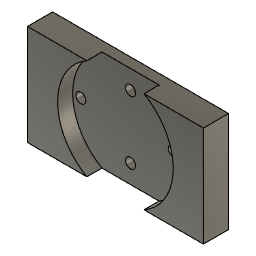
simple_mount v2 (Autodesk Fusion 360 design; units mm, degrees)
Autodesk Fusion 360 part; units mm, degrees
sketch "Sketch1" plane through (0, 0, 0) normal (0, 1, 0) x (1, 0, 0) in component "base_plate"
  line L0 (0, 0) -> (35, 0)
  line L1 (35, 0) -> (35, -20)
  line L2 (0, 0) -> (0, -20)
  line L3 (0, -20) -> (35, -20)
  dimension "d1" = 35
  dimension "d2" = 20
  dimension "d3" = 20
  constraint coincident L0.start L2.start
  constraint horizontal L0
  constraint perpendicular L0 L1
  constraint perpendicular L0 L2
  measures "d1" distance of L0.start L0.end
  measures "d2" distance of L0.end L1.end
  measures "d3" distance of L0.start L2.end
extrude "Extrude1" add sketch "Sketch1" along normal blind 5 in component "base_plate"
sketch "Sketch2" plane through (0, 0, 0) normal (0, -1, 0) x (1, 0, 0) in component "base_plate"
  line L0 (0, 20) -> (0, 0)
  line L1 (0, 0) -> (35, 0)
  line L2 (35, 0) -> (35, 20)
  line L3 (35, 20) -> (0, 20)
  line L4 (0, 10) -> (35, 10) construction
  line L5 (17.5, 20) -> (17.5, 0) construction
  circle A0 centre (7.6246, 10) radius 1
  circle A1 centre (26.0211, 10) radius 1
  dimension "d6" = 2
  dimension "d7" = 2
  constraint midpoint L0 L4.start
  constraint midpoint L2 L4.end
  constraint midpoint L3 L5.start
  constraint perpendicular L4 L5
  constraint coincident L4 A0.centre
  constraint coincident L4 A1.centre
  measures "d6" diameter of A0
  measures "d7" diameter of A1
extrude "Extrude2" cut sketch "Sketch2" against normal blind 5 contours A0 | A1 in component "base_plate"
sketch "Sketch3" plane through (0, 0, 0) normal (0, -1, 0) x (1, 0, 0) in component "base_plate"
  circle A0 centre (7.6246, 10) radius 1
  circle A1 centre (26.0211, 10) radius 1
  line L0 (0, 20) -> (0, 0)
  line L1 (0, 0) -> (35, 0)
  line L2 (35, 0) -> (35, 20)
  line L3 (35, 20) -> (0, 20)
  line L4 (17.5, 20) -> (17.5, 0) construction
  circle A2 centre (17.5, 16.2296) radius 1
  circle A3 centre (17.5, 3.7004) radius 1
  dimension "d10" = 2
  dimension "d11" = 2
  constraint midpoint L3 L4.start
  constraint midpoint L1 L4.end
  constraint coincident L4 A2.centre
  constraint coincident L4 A3.centre
  measures "d10" diameter of A2
  measures "d11" diameter of A3
extrude "Extrude3" cut sketch "Sketch3" against normal blind 5 contours A2 | A3 in component "base_plate"
sketch "Sketch4" plane through (0, 0, 0) normal (0, -1, 0) x (1, 0, 0) in component "base_plate"
  circle A0 centre (17.5, 3.7004) radius 1
  circle A1 centre (17.5, 16.2296) radius 1
  circle A2 centre (7.6246, 10) radius 1
  circle A3 centre (26.0211, 10) radius 1
  line L0 (0, 20) -> (0, 0)
  line L1 (0, 0) -> (35, 0)
  line L2 (35, 0) -> (35, 20)
  line L3 (35, 20) -> (0, 20)
  line L4 (17.5, 20) -> (17.5, 0) construction
  circle A4 centre (17.5, 10) radius 11.5
  constraint midpoint L3 L4.start
  constraint perpendicular L3 L4
  constraint midpoint L4 A4.centre
extrude "Extrude4" cut sketch "Sketch4" against normal blind 3 contours A0 | A1 | A2 | A3 | L1 L3 A4 in component "base_plate"
component "base_plate" placed x (1, 0, 0) y (0, 1, 0) z (0, 0, 1) at (0, 0, 0)
